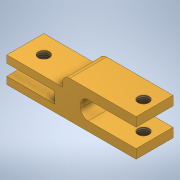
# Autodesk Inventor part: base_plate
Saved by Autodesk Inventor 2020 (Build 240168000, 168)
## iProperties
Created: 2020-03-15
Part Number: base_plate
Material: PC/ABS Plastic
Document SubType Name: Modeling
Designer: 0x6f736f646f
Density: 0.357273 g/cm^3
Appearance: Brass - Satin
Author: 0x6f736f646f
Autodesk Inventor part; units mm, degrees
ref_plane "YZ Plane" through (0, 0, 0) normal (1, 0, 0) x (0, 1, 0)
ref_plane "Work Plane1" through (0, 0, -25) normal (0, 0, 1) x (1, 0, 0)
sketch "Sketch4" plane through (0, 0, -25) normal (0, 0, 1) x (1, 0, 0)
  line L0 (70, -4.0026) -> (70, 3.9974)
  line L1 (72, 5.9974) -> (90, 5.9974)
  line L2 (90, 5.9974) -> (90, 3.4974)
  line L3 (90, 3.4974) -> (77, 3.4974)
  line L4 (75, 1.4974) -> (75, 0.4974)
  line L5 (77, -1.5026) -> (90, -1.5026)
  line L6 (90, -1.5026) -> (90, -4.0026)
  line L7 (90, -4.0026) -> (70, -4.0026)
  arc A0 (72, 5.9974) -> (70, 3.9974) centre (72, 3.9974) ccw
  arc A1 (77, 3.4974) -> (75, 1.4974) centre (77, 1.4974) ccw
  arc A2 (75, 0.4974) -> (77, -1.5026) centre (77, 0.4974) ccw
  line L8 (70, 0) -> (70, -3) projected
  line L9 (55, -4.0026) -> (55, -2.0026)
  line L10 (55, -2.0026) -> (68, -2.0026)
  line L11 (68, -2.0026) -> (68, 0.9974)
  line L12 (68, 0.9974) -> (55, 0.9974)
  line L13 (55, -4.0026) -> (70, -4.0026)
  line L14 (55, 0.9974) -> (55, 2.9974)
  line L15 (55, 2.9974) -> (70, 2.9974)
  point P0 (0, 0)
  dimension "d66" = 5
  dimension "d67" = 2.5
  dimension "d68" = 2.5
  dimension "d69" = 20
  dimension "d70" = 15
  dimension "d71" = 2
  dimension "d111" = 2
  dimension "d112" = 2
  dimension "d113" = 3
  dimension "d115" = 2
  dimension "d116" = 15
  dimension "d117" = 15
  constraints: 30 end point, 6 point on circle, 6 tangent, 5 perpendicular, 4 horizontal, 4 point on line, 3 centre point, 3 vertical, 2 equal radius, 1 parallel
  measures "d66" distance between parallel lines of L5 L3
  measures "d67" distance between parallel lines of L3 L1
  measures "d68" distance between parallel lines of L7 L5
  measures "d69" distance between parallel lines of L2 L0
  measures "d70" distance between parallel lines of L2 L4
  measures "d71" radius of A0
  measures "d111" distance between parallel lines of L13 L10
  measures "d112" distance between parallel lines of L0 L11
  measures "d113" distance between parallel lines of L10 L12
  measures "d115" distance between parallel lines of L12 L15
  measures "d116" distance between parallel lines of L0 L14
  measures "d117" distance between parallel lines of L0 L9
ref_plane "Work Plane5" through (72, 5.9974, -20) normal (0, 1, 0) x (1, 0, 0)
sketch "Sketch5" plane through (72, 5.9974, -20) normal (0, 1, 0) x (1, 0, 0)
  line L0 (18, 10) -> (18, 0) projected
  line L1 (0, 10) -> (18, 10) projected
  point P0 (-72, -20)
  point P1 (15, 5)
  dimension "d86" = 3
  dimension "d87" = 5
  measures "d86" distance from line of L0 point (15, 5)
  measures "d87" distance from line of point (15, 5) L1
hole "Hole1" [suppressed]
extrude "Extrusion5" add sketch "Sketch4" along normal mid plane 10
hole "Hole2" at (87, 5.9974, -25) direction (0, -1, 0) diameter 3 end through all
sketch "Sketch8" plane through (55, 2.9974, -20) normal (0, 1, 0) x (1, 0, 0)
  line L0 (0, 10) -> (15, 10) projected
  line L1 (0, 10) -> (0, 0) projected
  point P0 (-55, -20)
  point P1 (5, 5)
  dimension "d127" = 5
  dimension "d128" = 5
  measures "d127" distance from line of point (5, 5) L0
  measures "d128" distance from line of L1 point (5, 5)
hole "Hole3" at (60, 2.9974, -25) direction (0, -1, 0) diameter 3 end through all
thread "Thread1" size "M3x0.5" class "6H" standard "ANSI Metric M Profile" full length
thread "Thread2" size "M3x0.5" class "6H" standard "ANSI Metric M Profile" full length
thread "Thread3" size "M3x0.5" class "6H" standard "ANSI Metric M Profile" full length
thread "Thread4" size "M3x0.5" class "6H" standard "ANSI Metric M Profile" full length
body "Solid2"
